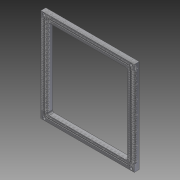
# Autodesk Inventor part: FlowChamberWalls
Saved by Autodesk Inventor 2011 (Build 150239000, 239)
## iProperties
Created: 2012-03-09
Part Number: FlowChamberWalls
Document SubType Name: Modeling
Designer: Marc
Density: 1 g/cm^3
Author: Marc
Autodesk Inventor part; units mm, degrees
ref_plane "YZ Plane" through (0, 0, 0) normal (1, 0, 0) x (0, 1, 0)
ref_plane "XZ Plane" through (0, 0, 0) normal (0, 1, 0) x (-1, 0, 0)
sketch "basic outline" plane through (0, 0, 0) normal (0, 0, 1) x (1, 0, 0)
  line L0 (-231.4919, 30.4572) -> (124.1081, 30.4572)
  line L1 (124.1081, 30.4572) -> (124.1081, -325.1428)
  line L2 (124.1081, -325.1428) -> (-231.4919, -325.1428)
  line L3 (-231.4919, -325.1428) -> (-231.4919, 30.4572)
  line L4 (-199.7419, 5.0572) -> (92.3581, 5.0572)
  line L5 (98.7081, -1.2928) -> (98.7081, -293.3928)
  line L6 (92.3581, -299.7428) -> (-199.7419, -299.7428)
  line L7 (-206.0919, -293.3928) -> (-206.0919, -1.2928)
  arc A0 (-206.0919, -293.3928) -> (-199.7419, -299.7428) centre (-199.7419, -293.3928) ccw
  arc A1 (92.3581, -299.7428) -> (98.7081, -293.3928) centre (92.3581, -293.3928) ccw
  arc A2 (98.7081, -1.2928) -> (92.3581, 5.0572) centre (92.3581, -1.2928) ccw
  arc A3 (-199.7419, 5.0572) -> (-206.0919, -1.2928) centre (-199.7419, -1.2928) ccw
  line L8 (-231.4919, -147.3428) -> (336.0603, -147.3428)
  line L9 (-53.6919, 30.4572) -> (-53.6919, -325.1428)
  point P0 (-206.0919, 5.0572)
  point P1 (98.7081, -299.7428)
  point P2 (98.7081, 5.0572)
  point P3 (124.1081, -147.3428)
  point P4 (98.7081, -147.3428)
  point P5 (-53.6919, 5.0572)
  point P6 (-53.6919, -299.7428)
  point P7 (-53.6919, -299.7428)
  point P8 (-206.0919, -147.3428)
  dimension "FlowChamber_OuterWidth" = 355.6
  dimension "FlowChamber_InnerWidth" = 304.8
  dimension "FlowChamber_InnerLength" = 304.8
  dimension "FlowChamber_InnerFillet" = 6.35
  dimension "FlowChamber_OuterLength" = 355.6
  constraints: 20 end point, 11 point on line, 9 midpoint, 8 point on circle, 8 tangent, 4 centre point, 4 parallel, 4 perpendicular, 3 equal radius, 2 horizontal
  measures "FlowChamber_OuterWidth" distance of L2.end L0.start
  measures "FlowChamber_InnerWidth" distance of point (98.708, 5.057) point (98.708, -299.743)
  measures "FlowChamber_InnerLength" distance of point (-206.092, 5.057) point (98.708, 5.057)
  measures "FlowChamber_InnerFillet" radius of A0
  measures "FlowChamber_OuterLength" distance of L1.end L2.end
extrude "frame" add sketch "basic outline" along normal blind 19.05 contours L0 L9 L4 A3 L7 L8 L3 | L0 L1 L8 L5 A2 L4 L9 | L8 L7 A0 L6 L9 L2 L3 | L1 L2 L9 L6 A1 L5 L8
sketch "Sketch2" plane through (0, 0, 19.05) normal (0, 0, 1) x (1, 0, 0)
  line L0 (-206.0919, -293.3928) -> (-206.0919, -1.2928) projected
  line L1 (-231.4919, -325.1428) -> (-231.4919, 30.4572) projected
  line L2 (-204.5174, 14.5822) -> (97.1336, 14.5822)
  line L3 (108.2331, 3.4827) -> (108.2331, -298.1683)
  line L4 (97.1336, -309.2678) -> (-204.5174, -309.2678)
  line L5 (-215.6169, -298.1683) -> (-215.6169, 3.4827)
  arc A0 (-204.5174, 14.5822) -> (-215.6169, 3.4827) centre (-204.5174, 3.4827) ccw
  arc A1 (-215.6169, -298.1683) -> (-204.5174, -309.2678) centre (-204.5174, -298.1683) ccw
  arc A2 (97.1336, -309.2678) -> (108.2331, -298.1683) centre (97.1336, -298.1683) ccw
  arc A3 (108.2331, 3.4827) -> (97.1336, 14.5822) centre (97.1336, 3.4827) ccw
  line L6 (-204.5174, 19.3822) -> (97.1336, 19.3822)
  line L7 (113.0331, 3.4827) -> (113.0331, -298.1683)
  line L8 (97.1336, -314.0678) -> (-204.5174, -314.0678)
  line L9 (-220.4169, -298.1683) -> (-220.4169, 3.4827)
  arc A4 (113.0331, 3.4827) -> (97.1336, 19.3822) centre (97.1336, 3.4827) ccw
  arc A5 (97.1336, -314.0678) -> (113.0331, -298.1683) centre (97.1336, -298.1683) ccw
  arc A6 (-220.4169, -298.1683) -> (-204.5174, -314.0678) centre (-204.5174, -298.1683) ccw
  arc A7 (-204.5174, 19.3822) -> (-220.4169, 3.4827) centre (-204.5174, 3.4827) ccw
  line L10 (-231.4919, -147.3428) -> (336.0603, -147.3428) projected
  line L11 (-53.6919, 30.4572) -> (-53.6919, -325.1428) projected
  point P0 (0, 0)
  point P1 (108.2331, -309.2678)
  point P2 (108.2331, 14.5822)
  point P3 (-215.6169, -309.2678)
  point P4 (-53.6919, 14.5822)
  point P5 (-215.6169, -147.3428)
  point P6 (113.0331, -314.0678)
  point P7 (113.0331, 19.3822)
  point P8 (-220.4169, -314.0678)
  point P9 (-220.4169, -147.3428)
  point P10 (-53.6919, -314.0678)
  point P11 (-53.6919, -309.2678)
  dimension "Oring_groove_length" = 323.85
  dimension "Oring_groove_width" = 323.85
  dimension "d12" = 11.0995
  dimension "d13" = 333.45
  dimension "d14" = 333.45
  dimension "d15" = 15.8995
  dimension "FlowChamber_inlet_thickness" = 25.4
  constraints: 16 end point, 16 point on circle, 16 point on line, 16 tangent, 8 centre point, 6 equal radius, 5 midpoint, 4 parallel, 2 horizontal, 2 perpendicular
  measures "Oring_groove_length" distance of point (108.233, -309.268) point (-215.617, -309.268)
  measures "Oring_groove_width" distance of point (108.233, 14.582) point (108.233, -309.268)
  measures "d12" radius of A0
  measures "d13" distance of point (113.033, -314.068) point (-220.417, -314.068)
  measures "d14" distance of point (113.033, 19.382) point (113.033, -314.068)
  measures "d15" radius of A4
  measures "FlowChamber_inlet_thickness" distance between parallel lines of L1 L0
extrude "top oring groove" cut sketch "Sketch2" against normal blind 2.7 contours A0 L5 L10 L9 A7 L6 L11 L2 | L11 L6 A4 L7 L10 L3 A3 L2 | L5 A1 L4 L11 L8 A6 L9 L10 | L10 L7 A5 L8 L11 L4 A2 L3
sketch "Sketch3" plane through (0, 0, 0) normal (0, 0, -1) x (-1, 0, 0)
  line L0 (215.6169, 3.4827) -> (215.6169, -298.1683) projected
  line L1 (220.4169, 3.4827) -> (220.4169, -298.1683) projected
  arc A0 (204.5174, -314.0678) -> (220.4169, -298.1683) centre (204.5174, -298.1683) ccw projected
  line L2 (204.5174, -309.2678) -> (-97.1336, -309.2678) projected
  line L3 (204.5174, -314.0678) -> (-97.1336, -314.0678) projected
  arc A1 (220.4169, 3.4827) -> (204.5174, 19.3822) centre (204.5174, 3.4827) ccw projected
  line L4 (-97.1336, 19.3822) -> (204.5174, 19.3822) projected
  arc A2 (-97.1336, 19.3822) -> (-113.0331, 3.4827) centre (-97.1336, 3.4827) ccw projected
  line L5 (-108.2331, -298.1683) -> (-108.2331, 3.4827) projected
  line L6 (-113.0331, -298.1683) -> (-113.0331, 3.4827) projected
  arc A3 (-113.0331, -298.1683) -> (-97.1336, -314.0678) centre (-97.1336, -298.1683) ccw projected
  arc A4 (-108.2331, -298.1683) -> (-97.1336, -309.2678) centre (-97.1336, -298.1683) ccw projected
  arc A5 (-97.1336, 14.5822) -> (-108.2331, 3.4827) centre (-97.1336, 3.4827) ccw projected
  line L7 (-97.1336, 14.5822) -> (204.5174, 14.5822) projected
  arc A6 (215.6169, 3.4827) -> (204.5174, 14.5822) centre (204.5174, 3.4827) ccw projected
  arc A7 (204.5174, -309.2678) -> (215.6169, -298.1683) centre (204.5174, -298.1683) ccw projected
  point P0 (0, 0)
  point P1 (220.4169, -314.0678)
extrude "bottom oring groove" cut sketch "Sketch3" against normal blind 2.7
sketch "Sketch4" plane through (0, 0, 0) normal (0, 0, -1) x (-1, 0, 0)
  line L0 (231.4919, -325.1428) -> (-124.1081, -325.1428) projected
  line L1 (204.5174, -314.0678) -> (-97.1336, -314.0678) projected
  line L2 (-113.0331, -298.1683) -> (-113.0331, 3.4827) projected
  line L3 (53.6919, 30.4572) -> (53.6919, -325.1428) projected
  line L4 (231.4919, -147.3428) -> (-336.0603, -147.3428) projected
  line L5 (-124.1081, -325.1428) -> (-124.1081, 30.4572) projected
  point P0 (0, 0)
  point P1 (-98.7081, -318.7928)
  point P2 (-47.9081, -318.7928)
  point P3 (2.8919, -318.7928)
  point P4 (53.6919, -318.7928)
  point P5 (104.4919, -318.7928)
  point P6 (155.2919, -318.7928)
  point P7 (206.0919, -318.7928)
  point P8 (-98.7081, 24.1072)
  point P9 (-47.9081, 24.1072)
  point P10 (2.8919, 24.1072)
  point P11 (53.6919, 24.1072)
  point P12 (104.4919, 24.1072)
  point P13 (155.2919, 24.1072)
  point P14 (206.0919, 24.1072)
  point P15 (-117.7581, -299.7428)
  point P16 (-117.7581, -248.9428)
  point P17 (-117.7581, -198.1428)
  point P18 (-117.7581, -147.3428)
  point P19 (-117.7581, -96.5428)
  point P20 (-117.7581, -45.7428)
  point P21 (-117.7581, 5.0572)
  point P22 (225.1419, -299.7428)
  point P23 (225.1419, -248.9428)
  point P24 (225.1419, -198.1428)
  point P25 (225.1419, -147.3428)
  point P26 (225.1419, -96.5428)
  point P27 (225.1419, -45.7428)
  point P28 (225.1419, 5.0572)
  dimension "d23" = 11.075
  dimension "HoldDownScrews_distFromEdge" = 6.35
  dimension "d27" = 50.8
  dimension "d32" = 342.9
  dimension "d80" = 6.35
  dimension "d83" = 50.8
  constraints: 16 symmetric about line, 1 horizontal, 1 vertical, 12 other
  measures "d23" distance from line of L0 L1.end
  measures "HoldDownScrews_distFromEdge" distance from line of L0 point (-98.708, -318.793)
  measures "d27" distance of point (-98.708, -318.793) point (-47.908, -318.793)
  measures "d32" distance of point (206.092, -318.793) point (206.092, 24.107)
  measures "d80" distance from line of L5 point (-117.758, -299.743)
  measures "d83" distance of point (-117.758, -299.743) point (-117.758, -248.943)
hole "hold down screws" at (98.7081, -318.7928, 0) at (47.9081, -318.7928, 0) at (-2.8919, -318.7928, 0) at (-53.6919, -318.7928, 0) at (-104.4919, -318.7928, 0) at (-155.2919, -318.7928, 0) at (-206.0919, -318.7928, 0) at (98.7081, 24.1072, 0) at (47.9081, 24.1072, 0) at (-2.8919, 24.1072, 0) at (-53.6919, 24.1072, 0) at (-104.4919, 24.1072, 0) at (-155.2919, 24.1072, 0) at (-206.0919, 24.1072, 0) at (-225.1419, 5.0572, 0) at (-225.1419, -45.7428, 0) at (-225.1419, -96.5428, 0) at (-225.1419, -147.3428, 0) at (-225.1419, -198.1428, 0) at (-225.1419, -248.9428, 0) at (-225.1419, -299.7428, 0) at (117.7581, -299.7428, 0) at (117.7581, -248.9428, 0) at (117.7581, -198.1428, 0) at (117.7581, -147.3428, 0) at (117.7581, -96.5428, 0) at (117.7581, -45.7428, 0) at (117.7581, 5.0572, 0) direction (0, 0, 1) diameter 2.159 depth 7.9375 tip angle 118
sketch "air port locations" plane through (-231.4919, -325.1428, 0) normal (-1, 0, 0) x (0, 0, 1)
  line L0 (19.05, 0) -> (19.05, 355.6) projected
  line L1 (0, 355.6) -> (0, 0) projected
  line L2 (19.05, 177.8) -> (0, 177.8)
  point P0 (0, 325.1428)
  point P1 (14.2875, 326.39)
  point P2 (14.2875, 318.77)
  point P3 (14.2875, 311.15)
  point P4 (14.2875, 303.53)
  point P5 (14.2875, 295.91)
  point P6 (14.2875, 288.29)
  point P7 (14.2875, 280.67)
  point P8 (14.2875, 273.05)
  point P9 (14.2875, 265.43)
  point P10 (14.2875, 257.81)
  point P11 (14.2875, 250.19)
  point P12 (14.2875, 242.57)
  point P13 (14.2875, 234.95)
  point P14 (14.2875, 227.33)
  point P15 (14.2875, 219.71)
  point P16 (14.2875, 212.09)
  point P17 (14.2875, 204.47)
  point P18 (14.2875, 196.85)
  point P19 (14.2875, 189.23)
  point P20 (14.2875, 181.61)
  point P21 (14.2875, 173.99)
  point P22 (14.2875, 166.37)
  point P23 (14.2875, 158.75)
  point P24 (14.2875, 151.13)
  point P25 (14.2875, 143.51)
  point P26 (14.2875, 135.89)
  point P27 (14.2875, 128.27)
  point P28 (14.2875, 120.65)
  point P29 (14.2875, 113.03)
  point P30 (14.2875, 105.41)
  point P31 (14.2875, 97.79)
  point P32 (14.2875, 90.17)
  point P33 (14.2875, 82.55)
  point P34 (14.2875, 74.93)
  point P35 (14.2875, 67.31)
  point P36 (14.2875, 59.69)
  point P37 (14.2875, 52.07)
  point P38 (14.2875, 44.45)
  point P39 (14.2875, 36.83)
  point P40 (14.2875, 29.21)
  dimension "portspacing" = 7.62
  dimension "TubeDistanceFromTop" = 4.7625
  constraints: 2 end point, 2 midpoint, 1 symmetric about line, 1 vertical, 39 other
  measures "portspacing" distance of point (14.288, 326.39) point (14.288, 318.77)
  measures "TubeDistanceFromTop" distance from line of L0 point (14.288, 29.21)
hole "10-32 flat bottom ports inlet" at (-231.4919, 1.2472, 14.2875) at (-231.4919, -6.3728, 14.2875) at (-231.4919, -13.9928, 14.2875) at (-231.4919, -21.6128, 14.2875) at (-231.4919, -29.2328, 14.2875) at (-231.4919, -36.8528, 14.2875) at (-231.4919, -44.4728, 14.2875) at (-231.4919, -52.0928, 14.2875) at (-231.4919, -59.7128, 14.2875) at (-231.4919, -67.3328, 14.2875) at (-231.4919, -74.9528, 14.2875) at (-231.4919, -82.5728, 14.2875) at (-231.4919, -90.1928, 14.2875) at (-231.4919, -97.8128, 14.2875) at (-231.4919, -105.4328, 14.2875) at (-231.4919, -113.0528, 14.2875) at (-231.4919, -120.6728, 14.2875) at (-231.4919, -128.2928, 14.2875) at (-231.4919, -135.9128, 14.2875) at (-231.4919, -143.5328, 14.2875) at (-231.4919, -151.1528, 14.2875) at (-231.4919, -158.7728, 14.2875) at (-231.4919, -166.3928, 14.2875) at (-231.4919, -174.0128, 14.2875) at (-231.4919, -181.6328, 14.2875) at (-231.4919, -189.2528, 14.2875) at (-231.4919, -196.8728, 14.2875) at (-231.4919, -204.4928, 14.2875) at (-231.4919, -212.1128, 14.2875) at (-231.4919, -219.7328, 14.2875) at (-231.4919, -227.3528, 14.2875) at (-231.4919, -234.9728, 14.2875) at (-231.4919, -242.5928, 14.2875) at (-231.4919, -250.2128, 14.2875) at (-231.4919, -257.8328, 14.2875) at (-231.4919, -265.4528, 14.2875) at (-231.4919, -273.0728, 14.2875) at (-231.4919, -280.6928, 14.2875) at (-231.4919, -288.3128, 14.2875) at (-231.4919, -295.9328, 14.2875) direction (1, 0, 0) diameter 3.9624 depth 6.604 countersink diameter 5.1054 countersink angle 90 thread size "10-32 UNF" class "2B" standard "ANSI Unified Screw Threads"
hole "air through holes inlet" at (-231.4919, 1.2472, 14.2875) at (-231.4919, -6.3728, 14.2875) at (-231.4919, -13.9928, 14.2875) at (-231.4919, -21.6128, 14.2875) at (-231.4919, -29.2328, 14.2875) at (-231.4919, -36.8528, 14.2875) at (-231.4919, -44.4728, 14.2875) at (-231.4919, -52.0928, 14.2875) at (-231.4919, -59.7128, 14.2875) at (-231.4919, -67.3328, 14.2875) at (-231.4919, -74.9528, 14.2875) at (-231.4919, -82.5728, 14.2875) at (-231.4919, -90.1928, 14.2875) at (-231.4919, -97.8128, 14.2875) at (-231.4919, -105.4328, 14.2875) at (-231.4919, -113.0528, 14.2875) at (-231.4919, -120.6728, 14.2875) at (-231.4919, -128.2928, 14.2875) at (-231.4919, -135.9128, 14.2875) at (-231.4919, -143.5328, 14.2875) at (-231.4919, -151.1528, 14.2875) at (-231.4919, -158.7728, 14.2875) at (-231.4919, -166.3928, 14.2875) at (-231.4919, -174.0128, 14.2875) at (-231.4919, -181.6328, 14.2875) at (-231.4919, -189.2528, 14.2875) at (-231.4919, -196.8728, 14.2875) at (-231.4919, -204.4928, 14.2875) at (-231.4919, -212.1128, 14.2875) at (-231.4919, -219.7328, 14.2875) at (-231.4919, -227.3528, 14.2875) at (-231.4919, -234.9728, 14.2875) at (-231.4919, -242.5928, 14.2875) at (-231.4919, -250.2128, 14.2875) at (-231.4919, -257.8328, 14.2875) at (-231.4919, -265.4528, 14.2875) at (-231.4919, -273.0728, 14.2875) at (-231.4919, -280.6928, 14.2875) at (-231.4919, -288.3128, 14.2875) at (-231.4919, -295.9328, 14.2875) direction (1, 0, 0) diameter 1.016 depth 38.1 tip angle 118
ref_plane "vertical midplane" through (-53.6919, -325.1428, 0) normal (-1, 0, 0) x (0, 0, 1)
mirror "Mirror1" about plane through (-53.6919, -325.1428, 0) normal (-1, 0, 0) of "10-32 flat bottom ports inlet", "air through holes inlet"
sketch "Sketch6" plane through (0, 0, 19.05) normal (0, 0, 1) x (1, 0, 0)
  line L0 (124.1081, -325.1428) -> (-231.4919, -325.1428) projected
  line L1 (-231.4919, -147.3428) -> (336.0603, -147.3428) projected
  line L2 (-53.6919, 30.4572) -> (-53.6919, -325.1428) projected
  line L3 (-218.7919, 22.8372) -> (111.4081, 22.8372)
  line L4 (111.4081, 22.8372) -> (111.4081, -317.5228)
  line L5 (111.4081, -317.5228) -> (-218.7919, -317.5228)
  line L6 (-218.7919, -317.5228) -> (-218.7919, 22.8372)
  point P0 (0, 0)
  dimension "d89" = 12.7
  dimension "d90" = 7.62
  constraints: 8 end point, 4 coincident, 2 parallel, 1 horizontal, 1 perpendicular, 2 other
  measures "d89" horizontal distance of L0.end L5.end
  measures "d90" distance from line of L0 L5.end
hole "Hole4" at (-218.7919, -317.5228, 19.05) at (-218.7919, 22.8372, 19.05) at (111.4081, 22.8372, 19.05) at (111.4081, -317.5228, 19.05) direction (0, 0, -1) diameter 6.7564 end through all counterbore diameter 11.1252 counterbore depth 9.525 clearance for "Socket Head Cap Screw" size "1/4" standard "Ansi Unified Screw Threads"
equation "\"d12\" = oring_groove_fillet"
equation "\"d13\" = Oring_groove_length + 2 * oring_width"
equation "\"d14\" = Oring_groove_width + 2 * oring_width"
equation "\"d15\" = oring_groove_fillet + oring_width"
equation "\"d19\" = oring_depth"
equation "\"d21\" = oring_depth"
equation "\"d80\" = HoldDownScrews_distFromEdge"
equation "\"oring_depth\" = 2.7"
equation "\"oring_width\" = 4.8"
equation "\"oring_id\" = 406.273"
equation "\"oring_groove_fillet\" = -1.8299 * oring_id + 1.16495 * Oring_groove_length + 1.16495 * Oring_groove_width"
body "Solid1"
